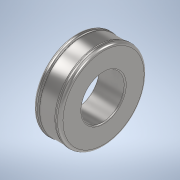
# Autodesk Inventor part: f8-16 thrust bearing
Saved by Autodesk Inventor 2020.4 (Build 244396000, 396)
## iProperties
Created: 2021-04-01
Part Number: f8-16 thrust bearing
Material: Stainless Steel
Document SubType Name: Modeling
Designer: AOB
Mass: 5.85737 g
Surface Area: 6.67408 cm^2
Volume: 0.732172 cm^3
Density: 8 g/cm^3
Appearance: Semi-Polished
Author: AOB
Autodesk Inventor part; units mm, degrees
ref_plane "YZ Plane" through (0, 0, 0) normal (1, 0, 0) x (0, 1, 0)
ref_plane "XZ Plane" through (0, 0, 0) normal (0, 1, 0) x (-1, 0, 0)
ref_plane "XY Plane" through (0, 0, 0) normal (0, 0, 1) x (1, 0, 0)
sketch "Sketch1" plane through (0, 0, 0) normal (0, 0, 1) x (1, 0, 0)
  line L0 (5, -0.5) -> (5, -3.8)
  line L1 (4.8, -4) -> (0.2, -4)
  line L2 (0, -3.8) -> (0, -0.5)
  arc A0 (0.5, 0) -> (0, -0.5) centre (0.5, -0.5) ccw
  arc A1 (5, -0.5) -> (4.5, 0) centre (4.5, -0.5) ccw
  line L3 (0.5, 0) -> (0.8, 0)
  line L4 (4.2, 0) -> (4.5, 0)
  arc A2 (1, -0.2) -> (0.8, 0) centre (0.8, -0.2) ccw
  arc A3 (4.2, 0) -> (4, -0.2) centre (4.2, -0.2) ccw
  line L5 (5, -4) -> (5, -8) construction
  line L6 (5, -8) -> (-0.4766, -8)
  line L7 (1.1, -0.1) -> (3.9, -0.1)
  line L8 (4, -0.2) -> (4, -0.2)
  arc A4 (4, -0.2) -> (3.9, -0.1) centre (3.9, -0.2) ccw
  line L9 (1, -0.2) -> (1, -0.2)
  arc A5 (1.1, -0.1) -> (1, -0.2) centre (1.1, -0.2) ccw
  arc A6 (4.8, -4) -> (5, -3.8) centre (4.8, -3.8) ccw
  arc A7 (0, -3.8) -> (0.2, -4) centre (0.2, -3.8) ccw
  point P0 (0, 0)
  point P1 (5, 0)
  point P2 (0, -4)
  point P3 (1.0268, -0.1)
  point P4 (3.9732, -0.1)
  point P5 (0.8978, 0)
  point P6 (0, -3.9)
  point P7 (0.1, -4)
  point P8 (5, -3.9)
  point P9 (4.9, -4)
  dimension "d0" = 5
  dimension "d1" = 4
  dimension "d2" = 0.5
  dimension "d4" = 0.2
  dimension "d5" = 4
  dimension "d9" = 0.1
  dimension "d10" = 0.1
  dimension "d13" = 0.2
  dimension "d14" = 0.2
  constraints: 20 end point, 17 point on circle, 14 point on line, 14 tangent, 8 centre point, 3 vertical, 2 equal radius, 2 perpendicular, 1 horizontal
  measures "d0" distance of point (0, 0) point (5, 0)
  measures "d1" distance of point (5, 0) L5.start
  measures "d2" radius of A0
  measures "d4" radius of A2
  measures "d5" distance of L5.start L5.end
  measures "d9" radius of A4
  measures "d10" radius of A5
  measures "d13" radius of A6
  measures "d14" radius of A7
revolve "Revolution1" add sketch "Sketch1" angle 360 about axis through (5, -8, 0) along (-1, 0, 0)
body "Solid1"
